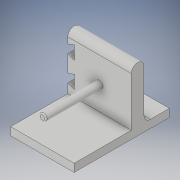
# Autodesk Inventor part: SpoolWinderBase
Saved by Autodesk Inventor 2019 (Build 230136000, 136)
## iProperties
Created: 2019-01-14
Part Number: SpoolWinderBase
Material: Generic
Document SubType Name: Modeling
Designer: Kepler
Density: 1 g/cm^3
Appearance: Default
Author: Kepler
Autodesk Inventor part; units mm, degrees
ref_plane "YZ Plane" through (0, 0, 0) normal (1, 0, 0) x (0, 1, 0)
ref_plane "XZ Plane" through (0, 0, 0) normal (0, 1, 0) x (-1, 0, 0)
ref_plane "XY Plane" through (0, 0, 0) normal (0, 0, 1) x (1, 0, 0)
sketch "Sketch1" plane through (0, 0, 0) normal (0, 0, 1) x (1, 0, 0)
  line L0 (0, 0) -> (50, 0)
  line L1 (50, 0) -> (50, 50)
  line L2 (50, 50) -> (0, 50)
  line L3 (0, 13.5853) -> (5.2, 11.6926)
  line L4 (5.2, 11.6926) -> (5.2, 22.0926)
  line L5 (5.2, 22.0926) -> (0, 20.2)
  line L6 (0, 50) -> (0, 20.2)
  line L7 (0, 13.5853) -> (0, 0)
  line L8 (0, 40.2) -> (5.2, 42.0926)
  line L9 (5.2, 42.0926) -> (5.2, 31.6926)
  line L10 (5.2, 31.6926) -> (0, 33.5853)
  dimension "d0" = 50
  dimension "d1" = 50
  dimension "d2" = 50
  dimension "d8" = 10.4
  dimension "d9" = 70
  dimension "d10" = 70
  dimension "d11" = 20.2
  dimension "d12" = 5.2
  dimension "d13" = 5.2
  dimension "d14" = 10.4
  dimension "d15" = 40.2
  dimension "d16" = 70
  dimension "d17" = 70
  dimension "d18" = 6.6147
  dimension "d19" = 6.6147
  dimension "d26" = 13.5853
  constraints: 22 end point, 4 perpendicular, 2 point on line, 2 vertical, 1 horizontal
  measures "d0" distance of L0.start L0.end
  measures "d1" distance of L0.end L1.end
  measures "d2" distance of L1.end L2.end
  measures "d8" distance of L3.end L4.end
  measures "d9" angle of L6 L5
  measures "d10" angle of L7 L3
  measures "d11" distance of L0.start L5.end
  measures "d12" distance from line of L6 L4.end
  measures "d13" distance from line of L6 L9.end
  measures "d14" distance of L8.end L9.end
  measures "d15" distance of L0.start L8.start
  measures "d16" angle of L6 L8
  measures "d17" angle of L6 L10
  measures "d18" distance of L10.end L8.start
  measures "d19" distance of L3.start L5.end
  measures "d26" distance of L0.start L3.start
extrude "Extrusion1" add sketch "Sketch1" along normal blind 10 contours L7 L3 L4 L5 L6 L10 L9 L8 L2 L1 L0
sketch "Sketch2" plane through (0, 0, 10) normal (0, 0, 1) x (1, 0, 0)
  line L0 (0, 13.5853) -> (0, 0) projected
  line L1 (0, 0) -> (50, 0)
  line L2 (50, 0) -> (50, 6.2593)
  line L3 (50, 0) -> (50, 50) projected
  line L4 (0, 0) -> (0, 6.2593)
  line L5 (0, 0) -> (50, 0) projected
  line L6 (0, 6.2593) -> (50, 6.2593)
  circle A0 centre (25, 25) radius 2.8
  dimension "d23" = 5.6
  constraints: 8 end point, 2 point on line, 1 centre point, 1 coincident, 1 collinear, 1 horizontal, 1 perpendicular
  measures "d23" diameter of A0
extrude "Extrusion2" add sketch "Sketch2" along normal blind 45
sketch "Sketch3" plane through (0, 0, 0) normal (0, 0, -1) x (-1, 0, 0)
  line L0 (0, 6.2593) -> (-50, 6.2593) projected
  line L1 (0, 6.2593) -> (-50, 6.2593)
  line L2 (0, 0) -> (-50, 0) projected
  line L3 (-50, 6.2593) -> (-50, 0)
  line L4 (-50, 0) -> (0, 0)
  line L5 (0, 6.2593) -> (0, 0) projected
  line L6 (0, 0) -> (0, 6.2593)
  constraints: 8 end point, 2 collinear, 2 perpendicular
extrude "Extrusion3" add sketch "Sketch3" along normal blind 20
fillet "Fillet1" radius 5 1 edges at (25, 6.2593, 0)
fillet "Fillet2" radius 5 1 edges at (25, 50, 0)
fillet "Fillet3" radius 5 1 edges at (25, 50, 10)
fillet "Fillet4" radius 1 1 edges at (22.2, 25, 55)
body "Solid1"
